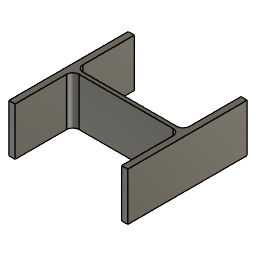
H-248×249×8×13 (Autodesk Fusion 360 design; units mm, degrees)
Autodesk Fusion 360 part; units mm, degrees
sketch "スケッチ1" plane through (0, 0, 0) normal (0, 0, 1) x (1, 0, 0)
  line L0 (0, 124.5) -> (0, -124.5)
  line L1 (248, -124.5) -> (248, 124.5)
  line L2 (235, -17) -> (235, -124.5)
  line L3 (13, -124.5) -> (13, -17)
  line L4 (0, -124.5) -> (13, -124.5)
  line L5 (235, -124.5) -> (248, -124.5)
  line L6 (222, 4) -> (26, 4)
  line L7 (26, -4) -> (222, -4)
  line L8 (13, 17) -> (13, 124.5)
  line L9 (13, 124.5) -> (0, 124.5)
  line L10 (235, 124.5) -> (235, 17)
  line L11 (248, 124.5) -> (235, 124.5)
  arc A0 (26, -4) -> (13, -17) centre (26, -17) ccw
  arc A1 (13, 17) -> (26, 4) centre (26, 17) ccw
  arc A2 (222, 4) -> (235, 17) centre (222, 17) ccw
  arc A3 (235, -17) -> (222, -4) centre (222, -17) ccw
extrude "押し出し1" add sketch "スケッチ1" along normal blind 100
